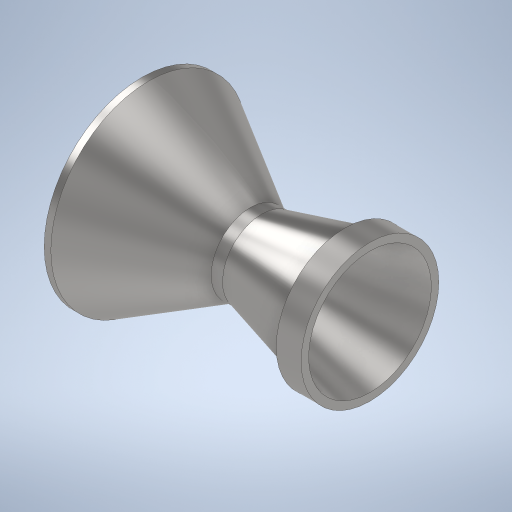
# Autodesk Inventor part: nozzle
Saved by Autodesk Inventor 2023 (Build 270158000, 158)
## iProperties
Created: 2022-09-14
Part Number: nozzle
Material: Stainless Steel, Austenitic
Document SubType Name: Modeling
Designer: station
Density: 8 g/cm^3
Appearance: Semi-Polished
Author: station
Autodesk Inventor part; units mm, degrees
ref_plane "YZ Plane" through (0, 0, 0) normal (1, 0, 0) x (0, 1, 0)
ref_plane "XZ Plane" through (0, 0, 0) normal (0, 1, 0) x (-1, 0, 0)
ref_plane "XY Plane" through (0, 0, 0) normal (0, 0, 1) x (1, 0, 0)
sketch "Sketch1" plane through (0, 0, 0) normal (0, 0, 1) x (1, 0, 0)
  line L0 (0, 0) -> (0, 54.375)
  line L1 (0, 54.375) -> (20, 54.375)
  line L2 (0, 0) -> (772.3927, 0)
  line L3 (253.9225, 18.624) -> (253.9225, 0) construction
  line L4 (192, 54.375) -> (253.9225, 18.624)
  line L5 (253.9225, 18.624) -> (256.9225, 18.624)
  line L6 (256.9225, 18.624) -> (325.3908, 36.97)
  line L7 (325.3908, 36.97) -> (325.3908, 0)
  line L8 (192, 54.375) -> (192, 0)
  line L9 (0, 54.375) -> (0, 74.375)
  line L10 (0, 74.375) -> (20, 74.375)
  line L11 (20, 74.375) -> (20, 58.375)
  line L12 (20, 58.375) -> (172, 58.375)
  line L13 (192, 54.375) -> (192, 74.375) construction
  line L14 (325.3908, 36.4995) -> (325.3908, 41.4995)
  line L15 (207, 50.3335) -> (253.2623, 23.624)
  line L16 (260.128, 23.624) -> (310.3908, 37.0919)
  line L17 (253.2623, 23.624) -> (260.128, 23.624)
  line L18 (310.3908, 41.4995) -> (310.3908, 37.0919)
  line L19 (207, 45.7147) -> (207, 21.1203)
  line L20 (325.3908, 36.4995) -> (325.3908, 41.4995)
  line L21 (325.3908, 41.4995) -> (310.3908, 41.4995)
  line L22 (207, 50.3335) -> (192, 58.9938)
  line L23 (207, 50.3335) -> (266.427, 50.3335) construction
  line L24 (172, 58.375) -> (185.0718, 58.375)
  line L25 (192, 58.9938) -> (188, 58.9938)
  line L26 (188, 58.9938) -> (188, 54.375)
  line L27 (188, 54.375) -> (192, 54.375)
  point P0 (255.4225, 18.624)
  dimension "d0" = 54.375
  dimension "d2" = 18.624
  dimension "d3" = 150
  dimension "d4" = 3
  dimension "d5" = 15
  dimension "d6" = 36.97
  dimension "d7" = 518.4701
  dimension "d8" = 20
  dimension "d9" = 20
  dimension "d10" = 16
  dimension "d18" = 4
  dimension "d21" = 5
  dimension "d22" = 15
  dimension "d23" = 150
  dimension "d24" = 4
  constraints: 56 end point, 9 perpendicular, 7 point on line, 4 horizontal, 2 vertical, 1 midpoint, 1 parallel
  measures "d0" distance of L0.start L1.start
  measures "d2" distance of L4.end L3.end
  measures "d3" angle of L4 L1
  measures "d4" distance of L4.end L5.end
  measures "d5" angle of L2 L6
  measures "d6" distance of L6.end L7.end
  measures "d7" distance from line of L2.end L3
  measures "d8" distance of L1.start L10.start
  measures "d9" distance of L10.start L11.start
  measures "d10" distance of L11.start L12.start
  measures "d18" distance between parallel lines of L4 L15
  measures "d21" distance of L14.end L14.start
  measures "d22" distance of L14.end L18.start
  measures "d23" angle of L23 L22
  measures "d24" distance of L22.end L25.end
revolve "Revolution1" add sketch "Sketch1" angle 360 about axis through (0, 0, 0) along (1, 0, 0) contours L27 L26 L25 L22 L15 L17 L16 L18 L21 L14 L6 L5 L4
body "Solid1"
